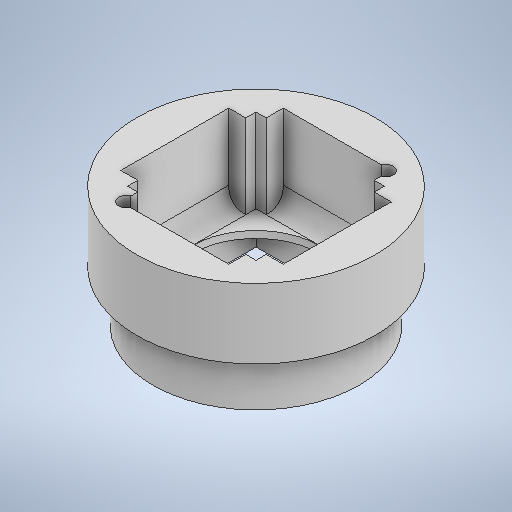
# Autodesk Inventor part: super flash light v4 head
Saved by Autodesk Inventor 2025 (Build 290162000, 162)
## iProperties
Created: 2024-06-28
Part Number: super flash light v4 head
Material: 一般
Document SubType Name: Modeling
Designer: gavin
Density: 1 g/cm^3
Appearance: 預設
Author: gavin
## iProperties of the stored document super flash light v4 head_3D 列印.ipt
Created: 2024-06-28
Part Number: super flash light v4 head_3D 列印
Material: 一般
Document SubType Name: Modeling
Designer: gavin
Density: 1 g/cm^3
Appearance: 預設
Author: gavin
Autodesk Inventor part; units mm, degrees
ref_plane "YZ Plane" through (0, 0, 0) normal (1, 0, 0) x (0, 1, 0)
ref_plane "XZ Plane" through (0, 0, 0) normal (0, 1, 0) x (-1, 0, 0)
ref_plane "XY Plane" through (0, 0, 0) normal (0, 0, 1) x (1, 0, 0)
sketch "草圖1" plane through (0, 0, 0) normal (0, 1, 0) x (-1, 0, 0)
  circle A0 centre (0, 0) radius 30.25
  circle A1 centre (0, 0) radius 34.95
  dimension "d0" = 60.5
  dimension "d1" = 4.7
  constraints: 2 centre point, 1 coincident
  measures "d0" diameter of A0
  measures "d1" radial gap between concentric circles of A0 A1
extrude "擠出1" add sketch "草圖1" against normal blind 15 contours A0
extrude "擠出2" add sketch "草圖1" along normal blind 20 contours A0 | A1
sketch "草圖3" plane through (0, 20, 0) normal (0, 1, 0) x (1, 0, 0)
  line L0 (-18.85, 18.85) -> (18.85, 18.85)
  line L1 (18.85, 18.85) -> (18.85, -18.85)
  line L2 (18.85, -18.85) -> (-18.85, -18.85)
  line L3 (-18.85, -18.85) -> (-18.85, 18.85)
  circle A0 centre (0, 0) radius 34.95 projected
  circle A1 centre (0, 0) radius 34.95 projected
  line L4 (-15.85, 18.85) -> (-15.85, 23.85)
  line L5 (-15.85, 23.85) -> (15.85, 23.85)
  line L6 (15.85, 23.85) -> (15.85, 18.85)
  line L7 (-18.85, -15.85) -> (-23.85, -15.85)
  line L8 (-23.85, -15.85) -> (-23.85, 15.85)
  line L9 (-23.85, 15.85) -> (-18.85, 15.85)
  line L10 (15.85, -18.85) -> (15.85, -23.85)
  line L11 (15.85, -23.85) -> (-15.85, -23.85)
  line L12 (-15.85, -23.85) -> (-15.85, -18.85)
  line L13 (18.85, 15.85) -> (23.85, 15.85)
  line L14 (23.85, 15.85) -> (23.85, -15.85)
  line L15 (23.85, -15.85) -> (18.85, -15.85)
  point P0 (-17.2304, -0.0475)
  dimension "d12" = 37.7
  dimension "d13" = 37.7
  dimension "d16" = 18.85
  dimension "d17" = 18.85
  dimension "d18" = 3
  dimension "d19" = 3
  dimension "d20" = 5
  constraints: 32 end point, 9 perpendicular, 2 parallel, 2 point on line, 1 horizontal, 1 vertical
  measures "d12" distance of L0.start L0.end
  measures "d13" distance of L0.end L1.end
  measures "d16" distance from line of A0.centre L1
  measures "d17" distance from line of A0.centre L0
  measures "d18" distance between parallel lines of L3 L4
  measures "d19" distance between parallel lines of L1 L6
  measures "d20" distance between parallel lines of L0 L5
extrude "擠出3" cut sketch "草圖3" against normal blind 24.1 contours L0 L1 L2 L3 | L4 L5 L6 L0 | L3 L7 L8 L9 | L13 L14 L15 L1 | L2 L10 L11 L12
fillet "圓角1" radius 5 1 edges at (0, -4.1, -23.85) curvature continuous yes
pattern_circular "環形陣列1" count 4 over 360 about axis through (0, -10, 0) along (0, 1, 0) of "圓角1"
sketch "草圖4" plane through (0, -4.1, 0) normal (0, 1, 0) x (1, 0, 0)
  circle A0 centre (0, 0) radius 18.85
  constraints: 1 centre point, 1 coincident
extrude "擠出4" cut sketch "草圖4" against normal up to surface (10.9 mm away)
sketch "草圖5" plane through (0, -15, 0) normal (0, -1, 0) x (1, 0, 0)
  line L0 (-20.01, 20.04) -> (20.04, 20.04)
  line L1 (20.04, 20.04) -> (20.04, -20.04)
  line L2 (20.04, -20.04) -> (-20.01, -20.04)
  line L3 (-20.01, -20.04) -> (-20.01, 20.04)
  point P0 (0, 0)
  dimension "d32" = 40.08
  dimension "d33" = 40.05
  dimension "d34" = 20.04
  dimension "d35" = 20.04
  constraints: 8 end point, 2 parallel, 1 horizontal, 1 perpendicular
  measures "d32" distance of L2.end L0.start
  measures "d33" distance of L0.start L0.end
  measures "d34" distance from line of point (0, 0) L1
  measures "d35" distance from line of point (0, 0) L0
extrude "擠出5" cut sketch "草圖5" against normal blind 8.9
sketch "草圖6" plane through (0, -15, 0) normal (0, -1, 0) x (1, 0, 0)
  circle A0 centre (15.0824, -22.9659) radius 2.25
  point P0 (0, 0)
  dimension "d38" = 4.5
  constraints: 1 centre point
  measures "d38" diameter of A0
extrude "擠出6" cut sketch "草圖6" against normal up to surface (35 mm away)
pattern_circular "環形陣列2" count 2 over 360 about axis through (0, -10, 0) along (0, 1, 0) of "擠出6"
thicken "增厚1" operation add thickness 0.5 both sides no extend neighbours no toward (0, 1, 0) faces at (-27.55, 20, 0)
